diaper guide (Autodesk Fusion 360 design; units mm, degrees)
Autodesk Fusion 360 part; units mm, degrees
sketch "Sketch1" plane through (0, 0, 0) normal (0, 0, 1) x (1, 0, 0)
  line L0 (0, 0) -> (30, 0)
  line L1 (30, 0) -> (30, 15)
  line L2 (30, 15) -> (0, 15)
  line L3 (0, 15) -> (0, 0)
  circle A0 centre (15, 7.5) radius 1
  line L4 (0, 0) -> (30, 0)
  line L5 (30, 0) -> (30, -5)
  line L6 (30, -5) -> (0, -5)
  line L7 (0, -5) -> (0, 0)
  dimension "d1" = 30
  dimension "d2" = 15
  dimension "d3" = 2
  dimension "d4" = 7.5
  dimension "d5" = 15
  dimension "d6" = 5
  constraint horizontal L0
  constraint vertical L1
  constraint horizontal L2
  constraint vertical L3
  constraint coincident L0.start L3.end
  constraint horizontal L4
  constraint vertical L5
  constraint horizontal L6
  constraint vertical L7
  measures "d1" distance of L0.start L0.end
  measures "d2" distance of L0.start L2.end
  measures "d3" diameter of A0
  measures "d4" distance of L2 A0.centre
  measures "d5" distance of L3 A0.centre
  measures "d6" distance of L0.end L5.end
extrude "Extrude1" add sketch "Sketch1" along normal blind 10
extrude "Extrude2" add sketch "Sketch1" against normal blind 15 contours L0 L4 L5 L6 L7
fillet "Fillet1" radius 3.5 2 edges at (15, 15, 10) (15, 15, 0)
